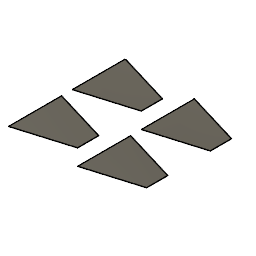
Contraction Chamber (Autodesk Fusion 360 design; units mm, degrees)
part number: 2025-11-29-13-42-13-855
Autodesk Fusion 360 part; units mm, degrees
sketch "Sketch1" plane through (0, 0, 0) normal (0, 0, 1) x (1, 0, 0)
  line L0 (-550, 550) -> (-550, 50)
  line L1 (-50, 400) -> (-50, 200)
  line L2 (-550, 550) -> (-50, 400)
  line L3 (-550, 50) -> (-50, 200)
  line L4 (-550, 50) -> (-50, 200)
  line L5 (-50, 400) -> (-50, 200)
  line L6 (-550, 550) -> (-50, 400)
  line L7 (-550, 550) -> (-550, 50)
  line L8 (-550, -50) -> (-550, -550)
  line L9 (-550, -50) -> (-50, -200)
  line L10 (-50, -200) -> (-50, -400)
  line L11 (-550, -550) -> (-50, -400)
  line L12 (100, -50) -> (600, -200)
  line L13 (100, -50) -> (100, -550)
  line L14 (100, -550) -> (600, -400)
  line L15 (600, -200) -> (600, -400)
  line L16 (600, 400) -> (600, 200)
  line L17 (100, 550) -> (600, 400)
  line L18 (100, 50) -> (600, 200)
  line L19 (100, 550) -> (100, 50)
  dimension "d1" = 500
  dimension "d2" = 200
  dimension "d5" = 500
  dimension "d6" = 200
  dimension "d7" = 500
  dimension "d8" = 500
  dimension "d9" = 200
  dimension "d10" = 500
  dimension "d11" = 500
  dimension "d12" = 200
  dimension "d13" = 500
  dimension "d14" = 500
  dimension "d15" = 200
  constraint vertical L0
  constraint parallel L0 L1
  constraint vertical L7
  constraint parallel L5 L7
  constraint vertical L8
  constraint vertical L13
  constraint vertical L19
  measures "d1" distance of L0.start L0.end
  measures "d2" distance of L1.start L1.end
  measures "d5" distance of L0.end L0.start
  measures "d6" distance of L1.end L1.start
  measures "d7" distance of L8.end L8.start
  measures "d8" distance of L8.end L8.start
  measures "d9" distance of L9.end L10.end
  measures "d10" distance of L13.end L12.start
  measures "d11" distance of L13.end L12.start
  measures "d12" distance of L14.end L12.end
  measures "d13" distance of L17.start L18.start
  measures "d14" distance of L17.start L18.start
  measures "d15" distance of L16.start L16.end
extrude "Extrude2" add sketch "Sketch1" along normal blind 2 makes body 1 at (-383.3333, -266.6667, 0) makes body 2 at (266.6667, -266.6667, 0) makes body 3 at (-383.3333, 333.3333, 0) makes body 4 at (266.6667, 333.3333, 0)
extrude "Extrude1" [suppressed]
